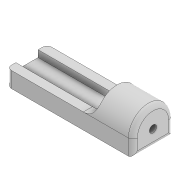
# Autodesk Inventor part: Cable_tie_connector_p2
Saved by Autodesk Inventor 2022 (Build 260153000, 153)
## iProperties
Created: 2022-07-19
Part Number: Cable_tie_connector_p2
Material: Generic
Document SubType Name: Modeling
Designer: dell
Density: 1 g/cm^3
Appearance: Default
Author: dell
Autodesk Inventor part; units mm, degrees
ref_plane "YZ Plane" through (0, 0, 0) normal (1, 0, 0) x (0, 1, 0)
ref_plane "XZ Plane" through (0, 0, 0) normal (0, 1, 0) x (-1, 0, 0)
ref_plane "XY Plane" through (0, 0, 0) normal (0, 0, 1) x (1, 0, 0)
sketch "Sketch1" plane through (0, 0, 0) normal (1, 0, 0) x (0, 1, 0)
  line L0 (3.5, 4.475) -> (0, 4.475)
  line L1 (0, 4.475) -> (0, -4.475)
  line L2 (0, -4.475) -> (3.5, -4.475)
  line L3 (3.5, -4.475) -> (3.5, -2.475)
  line L4 (3.5, -2.475) -> (2, -2.475)
  line L5 (2, -2.475) -> (2, 2.475)
  line L6 (2, 2.475) -> (3.5, 2.475)
  line L7 (3.5, 2.475) -> (3.5, 4.475)
  point P0 (0, 0)
  dimension "d0" = 2
  dimension "d1" = 2
  dimension "d2" = 2
  dimension "d4" = 2.475
  dimension "d5" = 2.475
  dimension "d6" = 1.5
  constraints: 16 end point, 7 perpendicular, 1 horizontal, 1 midpoint, 1 point on line
  measures "d0" distance between parallel lines of L1 L5
  measures "d1" distance between parallel lines of L0 L6
  measures "d2" distance between parallel lines of L2 L4
  measures "d4" distance from line of point (0, 0) L6
  measures "d5" distance from line of L4 point (0, 0)
  measures "d6" distance between parallel lines of L5 L7
extrude "Extrusion1" add sketch "Sketch1" along normal blind 20
sketch "Sketch2" plane through (20, 0, 0) normal (1, 0, 0) x (0, 0, -1)
  line L0 (-4.475, 0) -> (4.475, 0) projected
  line L1 (4.475, 0) -> (4.475, 3.5) projected
  line L2 (4.475, 3.5) -> (2.475, 3.5) projected
  line L3 (2.475, 3.5) -> (2.475, 2) projected
  line L4 (2.475, 2) -> (-2.475, 2) projected
  line L5 (-2.475, 2) -> (-2.475, 3.5) projected
  line L6 (-2.475, 3.5) -> (-4.475, 3.5) projected
  line L7 (-4.475, 3.5) -> (-4.475, 0) projected
  circle A0 centre (0, 3.5) radius 4.475
  line L8 (4.475, 0) -> (4.475, 3.5) projected
  point P0 (0, 0)
  point P1 (3.475, 3.5)
  point P2 (4.475, 3.5)
  point P3 (-4.475, 3.5)
  constraints: 2 tangent, 1 centre point, 1 horizontal alignment, 1 midpoint
extrude "Extrusion2" add sketch "Sketch2" along normal blind 8 contours L7 A0 L0 | A0 L6 L5 L4 L3 L2 L0 | A0 L2 L3 L4 L5 L6 | A0 L1 L0
sketch "Sketch3" plane through (20, 0, 0) normal (-1, 0, 0) x (0, 0, 1)
  circle A0 centre (0, 3.5) radius 0.8
  line L0 (-2.475, 2) -> (2.475, 2) projected
  line L1 (4.475, 0) -> (-4.475, 0) projected
  point P0 (0, 0)
  point P1 (0, 0)
  dimension "d11" = 1.6
  dimension "d17" = 1.5
  constraints: 1 centre point, 1 midpoint, 1 vertical alignment
  measures "d11" diameter of A0
  measures "d17" distance from line of L0 A0.centre
extrude "Extrusion3" cut sketch "Sketch3" against normal blind 10
fillet "Fillet1" radius 3 2 edges at (20, 3.5, 3.475) (20, 3.5, -3.475)
fillet "Fillet2" radius 1 4 edges at (28, 1.75, 4.475) (28, 1.75, -4.475) (28, 7.975, 0) (28, 0, 0)
fillet "Fillet3" radius 1 3 edges at (0, 0, 0) (0, 1.75, -4.475) (0, 1.75, 4.475)
body "Solid1"
